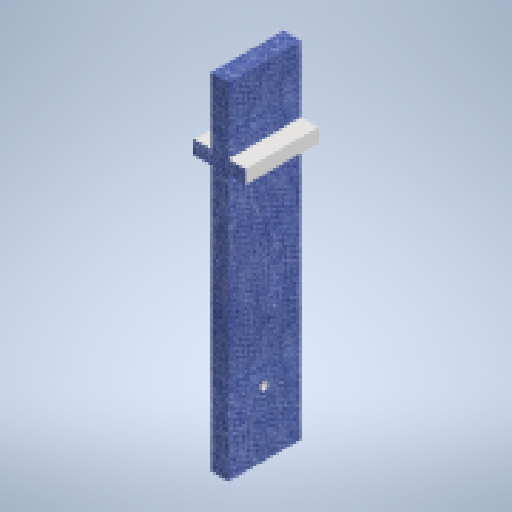
# Autodesk Inventor part: pared
Saved by Autodesk Inventor 2023 (Build 270158000, 158)
## iProperties
Created: 2024-08-02
Part Number: pared
Material: Generic
Document SubType Name: Modeling
Designer: sebas
Density: 1 g/cm^3
Appearance: Default
Author: sebas
Autodesk Inventor part; units mm, degrees
ref_plane "YZ Plane" through (0, 0, 0) normal (1, 0, 0) x (0, 1, 0)
ref_plane "XZ Plane" through (0, 0, 0) normal (0, 1, 0) x (-1, 0, 0)
ref_plane "XY Plane" through (0, 0, 0) normal (0, 0, 1) x (1, 0, 0)
sketch "Sketch1" plane through (0, 0, 0) normal (0, 1, 0) x (-1, 0, 0)
  line L0 (0, 0) -> (0, -42)
  line L1 (0, -42) -> (10, -42)
  line L2 (10, -42) -> (10, 0)
  line L3 (10, 0) -> (0, 0)
  dimension "d0" = 42
  dimension "d1" = 10
  dimension "d2" = 42
  constraints: 8 end point, 2 perpendicular, 1 vertical
  measures "d0" distance of L0.start L0.end
  measures "d1" distance of L0.end L1.end
  measures "d2" distance of L1.end L2.end
extrude "Extrusion1" add sketch "Sketch1" along normal blind 200
sketch "Sketch2" plane through (0, 0, 0) normal (1, 0, 0) x (0, 0, -1)
  line L0 (42, 200) -> (0, 200) projected
  line L1 (42, 200) -> (42, 161.5)
  line L2 (42, 0) -> (42, 200) projected
  line L3 (42, 161.5) -> (0, 161.5)
  line L4 (0, 0) -> (0, 200) projected
  line L5 (0, 161.5) -> (0, 153.5)
  line L6 (0, 153.5) -> (42, 153.5)
  line L7 (42, 153.5) -> (42, 161.5)
  dimension "d5" = 38.5
  dimension "d6" = 8
  constraints: 10 end point, 4 perpendicular, 3 point on line
  measures "d5" distance of L0.start L1.end
  measures "d6" distance of L3.end L5.end
extrude "Extrusion2" add sketch "Sketch2" along normal blind 10 contours L2 L6 L4 L3
sketch "Sketch3" plane through (-10, 0, -42) normal (-1, 0, 0) x (0, 0, 1)
  line L0 (42, 161.5) -> (42, 200) projected
  line L1 (42, 200) -> (42, 161.5)
  line L2 (42, 161.5) -> (0, 161.5)
  line L3 (0, 153.5) -> (42, 153.5) projected
  line L4 (0, 161.5) -> (0, 153.5)
  line L5 (42, 161.5) -> (42, 153.5) projected
  line L6 (0, 153.5) -> (42, 153.5)
  line L7 (42, 153.5) -> (42, 161.5)
  point P0 (42, 0)
  dimension "d9" = 38.5
  constraints: 10 end point, 3 perpendicular, 2 collinear
  measures "d9" distance of L0.end L0.start
extrude "Extrusion3" add sketch "Sketch3" along normal blind 10
sketch "Sketch4" plane through (-10, 0, -42) normal (-1, 0, 0) x (0, 0, 1)
  line L0 (42, 0) -> (42, 153.5) projected
  line L1 (42, 18.0001) -> (0, 57.4937)
  line L2 (0, 0) -> (0, 153.5) projected
  circle A0 centre (21, 37.7469) radius 2.65
  dimension "d12" = 5.3
  constraints: 2 end point, 2 point on line, 1 centre point, 1 midpoint
  measures "d12" diameter of A0
extrude "Extrusion4" cut sketch "Sketch4" against normal blind 10
body "Solid1"
